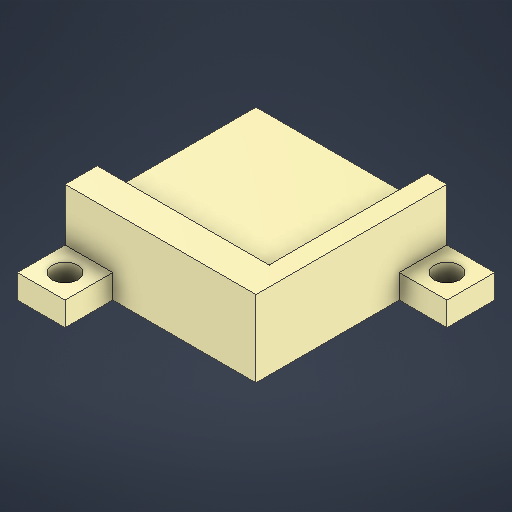
# Autodesk Inventor part: jetson_orin_nano_holder_corner
Saved by Autodesk Inventor 2026 (Build 300175050, 175E)
## iProperties
Created: 2025-06-11
Part Number: jetson_orin_nano_holder_corner
Material: Generic
Document SubType Name: Modeling
Designer: satom
Density: 1 g/cm^3
Appearance: Default
Author: satom
Autodesk Inventor part; units mm, degrees
ref_plane "YZ Plane" through (0, 0, 0) normal (1, 0, 0) x (0, 1, 0)
ref_plane "XZ Plane" through (0, 0, 0) normal (0, 1, 0) x (-1, 0, 0)
ref_plane "XY Plane" through (0, 0, 0) normal (0, 0, 1) x (1, 0, 0)
sketch "Sketch1" plane through (0, 0, 0) normal (0, 1, 0) x (-1, 0, 0)
  line L0 (0, 0) -> (96.52, 0)
  line L1 (96.52, 0) -> (96.52, -112.7)
  line L2 (96.52, -112.7) -> (0, -112.7)
  line L3 (0, -112.7) -> (0, 0)
  dimension "d0" = 96.52
  dimension "d1" = 112.7
  constraints: 8 end point, 2 parallel, 1 horizontal, 1 perpendicular
  measures "d0" distance of L0.start L0.end
  measures "d1" distance of L2.end L0.start
extrude "Extrusion1" add sketch "Sketch1" along normal blind 10.16
sketch "Sketch2" plane through (0, 10.16, 0) normal (0, 1, 0) x (1, 0, 0)
  line L0 (-96.52, 112.7) -> (-96.52, 0) construction
  line L1 (0, 0) -> (0, 112.7) construction
  line L2 (-96.52, 0) -> (0, 112.7) construction
  line L3 (0, 112.7) -> (-96.52, 112.7) construction
  line L4 (-96.52, 112.7) -> (0, 0) construction
  line L5 (-93.98, 4.28) -> (-2.54, 4.28)
  line L6 (-2.54, 4.28) -> (-2.54, 108.42)
  line L7 (-2.54, 108.42) -> (-93.98, 108.42)
  line L8 (-93.98, 108.42) -> (-93.98, 4.28)
  line L9 (-93.98, 4.28) -> (-2.54, 108.42) construction
  line L10 (-2.54, 4.28) -> (-93.98, 108.42) construction
  point P0 (-48.26, 56.35)
  dimension "d4" = 91.44
  dimension "d5" = 104.14
  constraints: 16 end point, 3 midpoint, 2 parallel, 1 horizontal, 1 perpendicular
  measures "d4" distance of L7.end L6.end
  measures "d5" distance of L5.end L6.end
extrude "Jetson Cavity" cut sketch "Sketch2" against normal blind 3.81
sketch "Sketch3" plane through (0, 0, 0) normal (0, -1, 0) x (1, 0, 0)
  line L0 (0, -19.05) -> (6.35, -19.05)
  line L1 (6.35, -19.05) -> (6.35, -25.4)
  line L2 (6.35, -25.4) -> (0, -25.4)
  circle A0 centre (3.175, -22.225) radius 1.7
  line L3 (6.35, -19.05) -> (0, -25.4) construction
  line L4 (-48.26, -112.7) -> (-48.26, 0) construction
  line L5 (-96.52, 0) -> (0, 0) construction
  line L6 (0, 0) -> (25.5083, 0) construction
  line L7 (6.35, -25.4) -> (0, -19.05) construction
  line L8 (-96.52, 0) -> (-96.52, -112.7) construction
  line L9 (0, -56.35) -> (-96.52, -56.35) construction
  line L10 (-96.52, -112.7) -> (-96.52, 0) construction
  line L11 (0, -19.05) -> (0, -25.4)
  line L12 (-96.52, -19.05) -> (-102.87, -19.05)
  line L13 (-102.87, -19.05) -> (-102.87, -25.4)
  line L14 (-102.87, -25.4) -> (-96.52, -25.4)
  circle A1 centre (-99.695, -22.225) radius 1.7
  line L15 (-102.87, -19.05) -> (-96.52, -25.4) construction
  line L16 (-102.87, -25.4) -> (-96.52, -19.05) construction
  line L17 (-96.52, -19.05) -> (-96.52, -25.4)
  line L18 (0, -93.65) -> (6.35, -93.65)
  line L19 (6.35, -93.65) -> (6.35, -87.3)
  line L20 (6.35, -87.3) -> (0, -87.3)
  circle A2 centre (3.175, -90.475) radius 1.7
  line L21 (6.35, -93.65) -> (0, -87.3) construction
  line L22 (6.35, -87.3) -> (0, -93.65) construction
  line L23 (0, -93.65) -> (0, -87.3)
  line L24 (-96.52, -93.65) -> (-102.87, -93.65)
  line L25 (-102.87, -93.65) -> (-102.87, -87.3)
  line L26 (-102.87, -87.3) -> (-96.52, -87.3)
  circle A3 centre (-99.695, -90.475) radius 1.7
  line L27 (-102.87, -93.65) -> (-96.52, -87.3) construction
  line L28 (-102.87, -87.3) -> (-96.52, -93.65) construction
  line L29 (-96.52, -93.65) -> (-96.52, -87.3)
  line L30 (0, 0) -> (0, -112.7) projected
  line L31 (-19.05, 0) -> (-25.4, 0)
  line L32 (-25.4, 0) -> (-25.4, 6.35)
  line L33 (-25.4, 6.35) -> (-19.05, 6.35)
  line L34 (-19.05, 6.35) -> (-19.05, 0)
  line L35 (-19.05, 0) -> (-25.4, 6.35) construction
  line L36 (-25.4, 0) -> (-19.05, 6.35) construction
  circle A4 centre (-22.225, 3.175) radius 1.7
  line L37 (0, 0) -> (-96.52, 0) construction
  line L38 (-77.47, 0) -> (-71.12, 0)
  line L39 (-71.12, 0) -> (-71.12, 6.35)
  line L40 (-71.12, 6.35) -> (-77.47, 6.35)
  line L41 (-77.47, 6.35) -> (-77.47, 0)
  line L42 (-77.47, 0) -> (-71.12, 6.35) construction
  line L43 (-71.12, 0) -> (-77.47, 6.35) construction
  circle A5 centre (-74.295, 3.175) radius 1.7
  line L44 (-96.52, -112.7) -> (0, -112.7) construction
  line L45 (-19.05, -112.7) -> (-25.4, -112.7)
  line L46 (-25.4, -112.7) -> (-25.4, -119.05)
  line L47 (-25.4, -119.05) -> (-19.05, -119.05)
  line L48 (-19.05, -119.05) -> (-19.05, -112.7)
  line L49 (-19.05, -112.7) -> (-25.4, -119.05) construction
  line L50 (-25.4, -112.7) -> (-19.05, -119.05) construction
  circle A6 centre (-22.225, -115.875) radius 1.7
  line L51 (0, -112.7) -> (-96.52, -112.7) construction
  line L52 (-77.47, -119.05) -> (-77.47, -112.7)
  line L53 (-71.12, -112.7) -> (-71.12, -119.05)
  line L54 (-71.12, -119.05) -> (-77.47, -119.05)
  line L55 (-77.47, -112.7) -> (-71.12, -119.05) construction
  line L56 (-71.12, -112.7) -> (-77.47, -119.05) construction
  line L57 (-77.47, -112.7) -> (-71.12, -112.7)
  circle A7 centre (-74.295, -115.875) radius 1.7
  dimension "d9" = 6.35
  dimension "d10" = 3.4
  dimension "d28" = 19.05
  dimension "d30" = 6.35
  dimension "d31" = 6.35
  dimension "d32" = 6.35
  dimension "d33" = 3.4
  dimension "d34" = 19.05
  constraints: 110 end point, 37 symmetric about line, 8 centre point, 4 midpoint, 4 point on line, 3 horizontal, 3 parallel, 3 perpendicular, 6 other
  measures "d9" distance of L0.end L1.end
  measures "d10" diameter of A0
  measures "d28" distance between parallel lines of L6 L0
  measures "d30" distance between parallel lines of L1 L30
  measures "d31" distance of L32.end L33.end
  measures "d32" distance of L31.end L32.end
  measures "d33" diameter of A4
  measures "d34" distance between parallel lines of L30 L34
extrude "Screws" add sketch "Sketch3" against normal blind 3.175
sketch "Sketch5" plane through (0, 0, 0) normal (0, -1, 0) x (1, 0, 0)
  line L0 (-96.52, 0) -> (0, 0) projected
  line L1 (0, 0) -> (0, -112.7) projected
  line L2 (-25.4, 6.35) -> (6.35, 6.35)
  line L3 (6.35, 6.35) -> (6.35, -25.4)
  line L4 (6.35, -25.4) -> (-25.4, -25.4)
  line L5 (-25.4, -25.4) -> (-25.4, 6.35)
  line L6 (-19.05, 6.35) -> (-25.4, 6.35) projected
  line L7 (6.35, -25.4) -> (6.35, -19.05) projected
  line L8 (6.35, 6.35) -> (-102.87, 6.35)
  line L9 (-102.87, 6.35) -> (-102.87, -119.05)
  line L10 (-102.87, -119.05) -> (6.35, -119.05)
  line L11 (6.35, -119.05) -> (6.35, 6.35)
  line L12 (-77.47, -119.05) -> (-71.12, -119.05) projected
  line L13 (-102.87, -87.3) -> (-102.87, -93.65) projected
  point P0 (6.35, -112.7)
  point P1 (0, -106.35)
  dimension "d35" = 25.4
  dimension "d37" = 25.4
  constraints: 16 end point, 4 collinear, 4 parallel, 2 horizontal, 2 perpendicular
  measures "d35" distance between parallel lines of L0 L4
  measures "d37" distance between parallel lines of L5 L1
extrude "Extrusion5" cut sketch "Sketch5" against normal through all contours L5 L4 L11 L10 L9 L8
equation "\"d10\" = m3_clearance"
equation "\"d33\" = m3_clearance"
equation "\"m3_heat_set_insert\" = 4"
equation "\"m3_clearance\" = 3.4"
equation "\"m3_heat_set_depth\" = 7"
equation "\"robot_diameter\" = 354"
equation "\"hardboard_thickness\" = 5"
body "Solid1"
